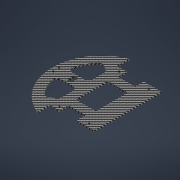
# Autodesk Inventor part: top
Saved by Autodesk Inventor 2022 (Build 260153000, 153)
## iProperties
Created: 2021-10-12
Part Number: top
Material: CFRP
Document SubType Name: Modeling
Designer: shiok
Density: 1.43 g/cm^3
Appearance: カーボンファイバー
Mass: 26.7457 g
Surface Area: 243.408 cm^2
Volume: 18.7033 cm^3
Author: shiok
Autodesk Inventor part; units mm, degrees
ref_plane "YZ Plane" through (0, 0, 0) normal (1, 0, 0) x (0, 1, 0)
ref_plane "XZ Plane" through (0, 0, 0) normal (0, 1, 0) x (-1, 0, 0)
ref_plane "XY Plane" through (0, 0, 0) normal (0, 0, 1) x (1, 0, 0)
sketch "スケッチ1" plane through (0, 0, 0) normal (0, 1, 0) x (-1, 0, 0)
  line L0 (62.5, 0) -> (-62.5, 0)
  line L1 (-10.5, -42.5) -> (-10.5, -31.5)
  line L2 (-10.5, -31.5) -> (10.5, -31.5)
  line L3 (10.5, -31.5) -> (10.5, -42.5)
  line L4 (0, -31.5) -> (0, -42.5)
  line L5 (0, 62.5) -> (0, -62.5)
  line L6 (-10.5, 42.5) -> (-10.5, 31.5)
  line L7 (-10.5, 31.5) -> (10.5, 31.5)
  line L8 (10.5, 31.5) -> (10.5, 42.5)
  line L9 (23, -42.5) -> (10.5, -42.5)
  line L10 (-10.5, -42.5) -> (-33, -42.5)
  line L11 (23, 58.1141) -> (23, 42.5)
  line L12 (23, -42.5) -> (23, -58.1141)
  line L13 (23, 42.5) -> (10.5, 42.5)
  arc A0 (23, -58.1141) -> (23, 58.1141) centre (0, 0) ccw
  arc A1 (23, 58.1141) -> (23, -58.1141) centre (0, 0) ccw construction
  line L14 (-33, 0) -> (-33, -42.5)
  line L15 (-10.5, 42.5) -> (-33, 42.5)
  line L16 (-33, 0) -> (-33, 42.5)
  point P0 (15.75, -37.5)
  point P1 (-21.75, -37.5)
  point P2 (15.75, 37.5)
  point P3 (-21.75, 37.5)
  point P4 (-23, -42.5)
  dimension "d1" = 37.5
  dimension "d2" = 21.75
  dimension "d4" = 37.5
  dimension "d8" = 21
  dimension "d25" = 63
  dimension "d27" = 23
  dimension "d30" = 62.5
  dimension "d32" = 11
  dimension "d48" = 42.5
  dimension "d50" = 22.5
  constraints: 34 end point, 8 point on circle, 8 symmetric about line, 4 midpoint, 3 point on line, 3 vertical, 2 centre point, 2 collinear, 1 coincident, 1 horizontal, 1 horizontal alignment, 1 parallel, 1 perpendicular
  measures "d1" distance of point (-21.75, -37.5) point (15.75, -37.5)
  measures "d2" horizontal distance of point (0, 0) point (-21.75, -37.5)
  measures "d4" vertical distance of point (0, 0) point (-21.75, -37.5)
  measures "d8" distance between parallel lines of L1 L3
  measures "d25" distance between parallel lines of L7 L2
  measures "d27" distance from line of L12 point (0, 0)
  measures "d30" radius of A0
  measures "d32" distance between parallel lines of L2 L9
  measures "d48" distance from line of L13 point (0, 0)
  measures "d50" distance between parallel lines of L1 L14
extrude "押し出し1" add sketch "スケッチ1" along normal blind 1.6
sketch "スケッチ2" plane through (0, 1.6, 0) normal (0, 1, 0) x (1, 0, 0)
  line L0 (62.5, 0) -> (-62.5, 0)
  point P0 (0, 0)
  point P1 (0, 0)
  point P2 (-15.75, 37.5)
  point P3 (21.75, 37.5)
  point P4 (0, 0)
  point P5 (21.75, -37.5)
  point P6 (-15.75, -37.5)
  dimension "d14" = 37.5
  dimension "d15" = 21.75
  dimension "d16" = 37.5
  constraints: 2 end point, 2 midpoint, 2 symmetric about line, 1 horizontal
  measures "d14" distance of point (21.75, 37.5) point (-15.75, 37.5)
  measures "d15" horizontal distance of point (0, 0) point (21.75, 37.5)
  measures "d16" vertical distance of point (0, 0) point (21.75, 37.5)
hole "穴1" at (21.75, 1.6, -37.5) at (-15.75, 1.6, -37.5) at (-15.75, 1.6, 37.5) at (21.75, 1.6, 37.5) direction (0, -1, 0) diameter 2.4 end through all clearance for "Countersunk Flat Head Screw ISO 2009/7046" size "M2" standard "ISO"
sketch "スケッチ3" plane through (0, 1.6, 0) normal (0, 1, 0) x (1, 0, 0)
  arc A0 (-23, 58.1141) -> (-23, -58.1141) centre (0, 0) ccw projected
  point P0 (-57.5, 3.75)
  point P1 (-57.5, -3.75)
  point P2 (-62.5, 0)
  dimension "d33" = 57.5
  dimension "d34" = 7.5
  dimension "d35" = 3.75
  constraints: 1 point on circle, 1 vertical alignment
  measures "d33" horizontal distance of point (0, 0) point (-57.5, -3.75)
  measures "d34" distance of point (-57.5, 3.75) point (-57.5, -3.75)
  measures "d35" vertical distance of point (0, 0) point (-57.5, -3.75)
hole "穴2" at (-57.5, 1.6, 3.75) at (-57.5, 1.6, -3.75) direction (0, -1, 0) diameter 2.4 depth 1.6 tip angle 118 clearance for "Countersunk Flat Head Screw ISO 2009/7046" size "M2" standard "ISO"
sketch "スケッチ4" plane through (0, 1.6, 0) normal (0, 1, 0) x (1, 0, 0)
  line L0 (-10.5, 20) -> (10.5, 20)
  line L1 (12.5, 18) -> (12.5, -18)
  line L2 (10.5, -20) -> (-10.5, -20)
  line L3 (-12.5, -18) -> (-12.5, 18)
  line L4 (-22.6562, 0) -> (23.8715, 0)
  line L5 (-12.5, 20) -> (12.5, -20) construction
  line L6 (12.5, 20) -> (-12.5, -20) construction
  arc A0 (-10.5, 20) -> (-12.5, 18) centre (-10.5, 18) ccw
  arc A1 (12.5, 18) -> (10.5, 20) centre (10.5, 18) ccw
  arc A2 (10.5, -20) -> (12.5, -18) centre (10.5, -18) ccw
  arc A3 (-12.5, -18) -> (-10.5, -20) centre (-10.5, -18) ccw
  point P0 (0, 0)
  point P1 (0, 0)
  dimension "d43" = 25
  dimension "d44" = 40
  dimension "d45" = 2
  constraints: 14 end point, 9 point on line, 8 point on circle, 8 tangent, 4 centre point, 3 equal radius, 3 midpoint, 2 horizontal, 2 parallel, 1 perpendicular
  measures "d43" distance of L5.start L6.start
  measures "d44" distance of L6.start L5.end
  measures "d45" radius of A0
extrude "押し出し2" cut sketch "スケッチ4" against normal up to surface (1.6 mm away)
sketch "スケッチ5" plane through (0, 1.6, 0) normal (0, 1, 0) x (1, 0, 0)
  arc A0 (-38.3634, 33.6043) -> (-49.0809, 13.8587) centre (0, 0) ccw
  line L0 (-12.5, -18) -> (-12.5, 18) projected
  line L1 (10.5, -20) -> (-10.5, -20) projected
  line L2 (-24, 26.7769) -> (-24, 12.5)
  arc A1 (-23, 58.1141) -> (-23, -58.1141) centre (0, 0) ccw projected
  line L3 (-10.5, 42.5) -> (-23, 42.5) construction
  arc A2 (-34.5, 42.5) -> (-23, 31) centre (-23, 42.5) ccw construction
  line L4 (-51, 0) -> (-24, 0)
  line L5 (-31.9353, 34.539) -> (-26.333, 31.0062)
  arc A3 (-49.0809, -13.8587) -> (-38.3634, -33.6043) centre (0, 0) ccw
  line L6 (-24, -26.7769) -> (-24, -12.5)
  line L7 (-31.9353, -34.539) -> (-26.333, -31.0062)
  line L8 (-44.2691, 7.5) -> (-29, 7.5)
  line L9 (-29, -7.5) -> (-44.2691, -7.5)
  arc A4 (-44.2691, -7.5) -> (-49.0809, -13.8587) centre (-44.2691, -12.5) ccw
  arc A5 (-49.0809, 13.8587) -> (-44.2691, 7.5) centre (-44.2691, 12.5) ccw
  arc A6 (-24, -12.5) -> (-29, -7.5) centre (-29, -12.5) ccw
  arc A7 (-26.333, -31.0062) -> (-24, -26.7769) centre (-29, -26.7769) ccw
  arc A8 (-38.3634, -33.6043) -> (-31.9353, -34.539) centre (-34.6023, -30.3097) ccw
  arc A9 (-29, 7.5) -> (-24, 12.5) centre (-29, 12.5) ccw
  arc A10 (-24, 26.7769) -> (-26.333, 31.0062) centre (-29, 26.7769) ccw
  arc A11 (-31.9353, 34.539) -> (-38.3634, 33.6043) centre (-34.6023, 30.3097) ccw
  line L10 (-37.1345, 5) -> (-36.1345, 5)
  line L11 (-34.1345, 3) -> (-34.1345, -3)
  line L12 (-36.1345, -5) -> (-37.1345, -5)
  line L13 (-39.1345, -3) -> (-39.1345, 3)
  line L14 (-44.2691, 12.5) -> (-29, 12.5) construction
  line L15 (-44.2691, -12.5) -> (-29, -12.5) construction
  line L16 (-36.6345, -12.5) -> (-36.6345, 12.5) construction
  arc A12 (-37.1345, 5) -> (-39.1345, 3) centre (-37.1345, 3) ccw
  arc A13 (-34.1345, 3) -> (-36.1345, 5) centre (-36.1345, 3) ccw
  arc A14 (-36.1345, -5) -> (-34.1345, -3) centre (-36.1345, -3) ccw
  arc A15 (-39.1345, -3) -> (-37.1345, -5) centre (-37.1345, -3) ccw
  point P0 (-35.3931, 36.7196)
  point P1 (-24, 29.535)
  point P2 (-29.1341, 32.7726)
  point P3 (-35.3931, -36.7196)
  point P4 (-24, -29.535)
  point P5 (-50.4455, 7.5)
  point P6 (-24, 7.5)
  point P7 (-24, -7.5)
  point P8 (-50.4455, -7.5)
  point P9 (-24, 7.5)
  point P10 (-34.1345, -5)
  point P11 (-34.1345, 5)
  point P12 (-39.1345, -5)
  dimension "d51" = 11.5
  dimension "d52" = 11.5
  dimension "d53" = 11.5
  dimension "d58" = 15
  dimension "d59" = 5
  dimension "d60" = 2.5
  dimension "d61" = 5
  dimension "d63" = 2
  constraints: 37 point on circle, 28 end point, 25 tangent, 21 point on line, 15 centre point, 10 equal radius, 4 horizontal, 4 parallel, 3 midpoint, 2 perpendicular, 2 symmetric about line, 1 coincident, 4 other
  measures "d51" distance between parallel lines of L0 L2
  measures "d52" radial gap between concentric circles of A1 A0
  measures "d53" radius of A2
  measures "d58" distance between parallel lines of L8 L9
  measures "d59" radius of A4
  measures "d60" distance between parallel lines of L9 L12
  measures "d61" distance between parallel lines of L11 L13
  measures "d63" radius of A12
extrude "押し出し3" cut sketch "スケッチ5" against normal blind 5
